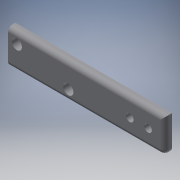
# Autodesk Inventor part: Chain_drag
Saved by Autodesk Inventor 2019.3 (Build 233278000, 278)
## iProperties
Created: 2020-09-10
Part Number: Chain_drag
Material: Generisch
Document SubType Name: Modeling
Designer: Nicolas Frick
Density: 1 g/cm^3
Appearance: Vorgabe
Author: Nicolas Frick
Autodesk Inventor part; units mm, degrees
ref_plane "YZ Plane" through (0, 0, 0) normal (1, 0, 0) x (0, 1, 0)
ref_plane "XZ Plane" through (0, 0, 0) normal (0, 1, 0) x (-1, 0, 0)
ref_plane "XY Plane" through (0, 0, 0) normal (0, 0, 1) x (1, 0, 0)
sketch "Skizze1" plane through (0, 0, 0) normal (0, 0, 1) x (1, 0, 0)
  line L0 (-4.2593, -15) -> (-4.2593, 15) construction
  line L1 (-4.2593, -15) -> (4.6613, -15) construction
  arc A0 (71.1407, -18.3849) -> (4.6613, -15) centre (32.8959, -114.9901) ccw construction
  line L2 (71.1407, -12.6613) -> (71.1407, -18.3849) construction
  line L3 (72.2593, -12.6613) -> (71.1407, -12.6613) construction
  line L4 (72.2593, -19) -> (72.2593, -12.6613) construction
  line L5 (75.2593, -19) -> (72.2593, -19) construction
  line L6 (75.2593, -9.9704) -> (75.2593, -19) construction
  arc A1 (75.2593, -9.9704) -> (13.1677, 13.0021) centre (8.1722, -95.8991) ccw construction
  arc A2 (11.2593, 15) -> (13.1677, 13.0021) centre (13.2593, 15) ccw construction
  line L7 (11.2593, 15) -> (-4.2593, 15) construction
  arc A3 (7.8907, 11.0161) -> (3.5907, 11.0161) centre (5.7407, 11.0161) ccw construction
  line L8 (7.8907, 6.0161) -> (7.8907, 11.0161) construction
  arc A4 (3.5907, 6.0161) -> (7.8907, 6.0161) centre (5.7407, 6.0161) ccw construction
  line L9 (3.5907, 11.0161) -> (3.5907, 6.0161) construction
  line L10 (7.8907, -10.5786) -> (7.8907, -5.5786) construction
  arc A5 (3.5907, -10.5786) -> (7.8907, -10.5786) centre (5.7407, -10.5786) ccw construction
  line L11 (3.5907, -5.5786) -> (3.5907, -10.5786) construction
  arc A6 (7.8907, -5.5786) -> (3.5907, -5.5786) centre (5.7407, -5.5786) ccw construction
  arc A7 (77.2593, -11.57) -> (68.4849, -5.0872) centre (8.1722, -95.8991) ccw construction
  arc A8 (68.4849, -5.0872) -> (68.1407, -6.2089) centre (70.1407, -6.2089) ccw construction
  line L12 (68.1407, -19.3793) -> (68.1407, -6.2089) construction
  arc A9 (71.1407, -20.5393) -> (68.1407, -19.3793) centre (32.8959, -114.9901) ccw construction
  line L13 (71.1407, -13) -> (71.1407, -20.5393) construction
  line L14 (73.1277, -13) -> (71.1407, -13) construction
  line L15 (73.1277, -21) -> (73.1277, -13) construction
  line L16 (77.2593, -21) -> (73.1277, -21) construction
  line L17 (77.2593, -11.57) -> (77.2593, -21) construction
  arc A10 (67.1407, -2.4739) -> (65.1407, -4.4739) centre (67.1407, -4.4739) ccw construction
  line L18 (67.1407, -2.4739) -> (68.1407, -2.4739) construction
  line L19 (68.1407, -2.4739) -> (68.1407, -14.8476) construction
  line L20 (22.4305, -2.4739) -> (87.7065, -2.4739)
  line L21 (87.7065, -2.4739) -> (87.7065, 11.9632)
  line L22 (87.7065, 11.9632) -> (22.4305, 11.9632)
  line L23 (22.4305, 11.9632) -> (22.4305, -2.4739)
  line L24 (26.0799, -2.4739) -> (26.0799, 7.5261) construction
  line L25 (47.5033, 11.9632) -> (47.5033, 1.9632) construction
  circle A11 centre (26.0799, 7.5261) radius 2.15
  circle A12 centre (47.5033, 1.9632) radius 2.15
  point P0 (0, 0)
  dimension "d0" = 10
  dimension "d1" = 10
  dimension "d2" = 4.3
  dimension "d3" = 4.3
  constraints: 12 end point, 3 perpendicular, 2 centre point, 2 coincident, 2 parallel, 2 point on line, 1 horizontal
  measures "d0" distance of L24.start L24.end
  measures "d1" distance of L25.start L25.end
  measures "d2" diameter of A11
  measures "d3" diameter of A12
extrude "Extrusion1" add sketch "Skizze1" along normal blind 3
sketch "Skizze2" plane through (0, 0, 0) normal (0, 0, -1) x (-1, 0, 0)
  arc A0 (-72.5805, 2.9132) -> (-72.5805, 6.2132) centre (-72.5805, 4.5632) ccw construction
  arc A1 (-73.5805, 6.2132) -> (-73.5805, 2.9132) centre (-73.5805, 4.5632) ccw construction
  arc A2 (-80.2805, 2.9132) -> (-80.2805, 6.2132) centre (-80.2805, 4.5632) ccw construction
  arc A3 (-81.2805, 6.2132) -> (-81.2805, 2.9132) centre (-81.2805, 4.5632) ccw construction
  circle A4 centre (-73.1179, 4.5632) radius 1.6
  circle A5 centre (-80.7335, 4.5632) radius 1.6
  point P0 (0, 0)
  dimension "d6" = 3.2
  dimension "d7" = 3.2
  constraints: 2 centre point
  measures "d6" diameter of A4
  measures "d7" diameter of A5
extrude "Extrusion2" cut sketch "Skizze2" against normal through all
fillet "Rundung1" radius 2 2 edges at (55.0685, 11.9632, 3) (87.7065, 4.7446, 3)
fillet "Rundung2" radius 2 3 edges at (87.1208, -2.4739, 2.4142) (87.7065, -2.4739, 0.5) (54.0685, -2.4739, 3)
